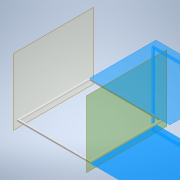
# Autodesk Inventor part: HoneyComb Frame
Saved by Autodesk Inventor 2022 (Build 260153000, 153)
## iProperties
Created: 2022-03-06
Part Number: HoneyComb Frame
Material: Generic
Document SubType Name: Modeling
Designer: calvi
Density: 1 g/cm^3
Appearance: Default
Author: calvi
Autodesk Inventor part; units mm, degrees
ref_plane "YZ Plane" through (0, 0, 0) normal (1, 0, 0) x (0, 1, 0)
ref_plane "XZ Plane" through (0, 0, 0) normal (0, 1, 0) x (-1, 0, 0)
ref_plane "XY Plane" through (0, 0, 0) normal (0, 0, 1) x (1, 0, 0)
ref_plane "Work Plane1" through (-1.5, 0, 1210) normal (-1, 0, 0) x (0, 0, 1)
sketch "Sketch1" plane through (-1.5, 0, 1210) normal (-1, 0, 0) x (0, 0, 1)
  circle A0 centre (-606.5, 339) radius 1.5 projected
  circle A1 centre (-848.5, 64) radius 1.5 projected
  circle A2 centre (-1090.5, 339) radius 1.5 projected
  circle A3 centre (-848.5, 614) radius 1.5 projected
  circle A4 centre (-364.5, 614) radius 1.5 projected
  circle A5 centre (-364.5, 64) radius 1.5 projected
  circle A6 centre (-122.5, 339) radius 1.5 projected
  circle A7 centre (-122.5, 614) radius 1.5 projected
  circle A8 centre (-122.5, 64) radius 1.5 projected
  circle A9 centre (-364.5, 339) radius 1.5 projected
  circle A10 centre (-606.5, 614) radius 1.5 projected
  circle A11 centre (-1090.5, 614) radius 1.5 projected
  circle A12 centre (-1090.5, 64) radius 1.5 projected
  circle A13 centre (-848.5, 339) radius 1.5 projected
  circle A14 centre (-606.5, 64) radius 1.5 projected
  line L0 (-1211.5, 0) -> (0, 0) projected
  line L1 (0, 0) -> (0, 1000) projected
  line L2 (-1211.5, 1000) -> (0, 1000) projected
  line L3 (-1211.5, 0) -> (-1211.5, 1000) projected
  line L4 (-25, 76.5) -> (-1186.5, 76.5)
  line L5 (-1186.5, 76.5) -> (-1186.5, 51.5)
  line L6 (-1186.5, 51.5) -> (-25, 51.5)
  line L7 (-25, 51.5) -> (-25, 76.5)
  line L8 (-122.5, 64) -> (-114.6022, 64)
  point P0 (-1210, 0)
  dimension "d0" = 25
  dimension "d1" = 25
  dimension "d2" = 25
  constraints: 10 end point, 2 horizontal, 2 parallel, 1 perpendicular, 1 other
  measures "d0" distance between parallel lines of L6 L4
  measures "d1" distance between parallel lines of L1 L7
  measures "d2" distance between parallel lines of L3 L5
ref_plane "Work Plane2" through (-1211.5, 0, -1.5) normal (1, 0, 0) x (0, 0, -1)
sketch "Sketch2" plane through (-1211.5, 0, -1.5) normal (1, 0, 0) x (0, 0, -1)
  line L0 (-25, 51.5) -> (-1186.5, 51.5) projected
  line L1 (-25, 76.5) -> (-25, 51.5) projected
  line L2 (-1186.5, 76.5) -> (-25, 76.5) projected
  line L3 (-1186.5, 51.5) -> (-1186.5, 76.5) projected
  circle A0 centre (-121, 64) radius 1.5 projected
  circle A1 centre (-363, 64) radius 1.5 projected
  circle A2 centre (-605, 64) radius 1.5 projected
  circle A3 centre (-847, 64) radius 1.5 projected
  circle A4 centre (-1089, 64) radius 1.5 projected
  point P0 (-1.5, 0)
extrude "Extrusion1" add sketch "Sketch2" along normal blind 25
extrude "Extrusion2" add sketch "Sketch1" along normal blind 25 contours L7 L6 L5 L4
ref_plane "Work Plane3" through (-1.5, 0, 1210) normal (-1, 0, 0) x (0, 0, 1)
sketch "Sketch3" plane through (-1.5, 0, 1210) normal (-1, 0, 0) x (0, 0, 1)
  line L0 (-1186.5, 76.5) -> (-1186.5, 51.5) projected
  line L1 (-1186.5, 51.5) -> (-1210, 51.5)
  line L2 (-1210, 51.5) -> (-1210, 76.5)
  line L3 (-1210, 76.5) -> (-1186.5, 76.5)
  line L4 (-1186.5, 76.5) -> (-1186.5, 51.5)
  line L5 (-1.5, 0) -> (-1.5, 1000) projected
  line L6 (-25, 76.5) -> (-25, 51.5) projected
  line L7 (-25, 51.5) -> (-1.5, 51.5)
  line L8 (-1.5, 51.5) -> (-1.5, 76.5)
  line L9 (-1.5, 76.5) -> (-25, 76.5)
  line L10 (-25, 76.5) -> (-25, 51.5)
  point P0 (-1210, 0)
  constraints: 16 end point, 4 parallel, 2 horizontal, 2 perpendicular, 1 point on line
extrude "Extrusion3" add sketch "Sketch3" along normal up to surface (1210 mm away)
sketch "Sketch4" plane through (-1.5, 51.5, 1208.5) normal (0, 0, 1) x (1, 0, 0)
  circle A0 centre (-121, 12.5) radius 1.5 projected
  circle A1 centre (-363, 12.5) radius 1.5 projected
  circle A2 centre (-605, 12.5) radius 1.5 projected
  circle A3 centre (-847, 12.5) radius 1.5 projected
  circle A4 centre (-1089, 12.5) radius 1.5 projected
  point P0 (1.5, -51.5)
hole "Hole1" at (-122.5, 64, 1208.5) at (-606.5, 64, 1208.5) at (-364.5, 64, 1208.5) at (-848.5, 64, 1208.5) at (-1090.5, 64, 1208.5) direction (0, 0, -1) diameter 3 end through all
body "Solid1"
